Autodesk Inventor part; units mm, degrees
(part 2 of 4)
  spline S77 degree 3 poles (0.8273, -16.5454) (1.5125, -16.5454) (2.0682, -15.9899) (2.0682, -15.3045) knots 2 2 2 2 3 3 3 3
  line L679 (0.8273, -16.5454) -> (1.5125, -16.5454) construction
  line L680 (1.5125, -16.5454) -> (2.0682, -15.9899) construction
  line L681 (2.0682, -15.9899) -> (2.0682, -15.3045) construction
  line L682 (2.0682, -15.3045) -> (2.0682, -9.5136)
  spline S78 degree 3 poles (2.0682, -9.5136) (2.0682, -8.8282) (1.5125, -8.2727) (0.8273, -8.2727) knots 4 4 4 4 5 5 5 5
  line L683 (2.0682, -9.5136) -> (2.0682, -8.8282) construction
  line L684 (2.0682, -8.8282) -> (1.5125, -8.2727) construction
  line L685 (1.5125, -8.2727) -> (0.8273, -8.2727) construction
  line L686 (0.8273, -8.2727) -> (-0.8273, -8.2727)
  spline S79 degree 3 poles (-0.8273, -8.2727) (-1.5127, -8.2727) (-2.0682, -8.8282) (-2.0682, -9.5136) knots 6 6 6 6 7 7 7 7
  line L687 (-0.8273, -8.2727) -> (-1.5127, -8.2727) construction
  line L688 (-1.5127, -8.2727) -> (-2.0682, -8.8282) construction
  line L689 (-2.0682, -8.8282) -> (-2.0682, -9.5136) construction
  line L690 (-2.0682, -9.5136) -> (-2.0682, -15.3045)
  spline S80 degree 3 poles (-2.0682, -27.7134) (-2.0682, -28.399) (-1.5127, -28.9543) (-0.8273, -28.9543) knots 0 0 0 0 1 1 1 1
  line L691 (-2.0682, -27.7134) -> (-2.0682, -28.399) construction
  line L692 (-2.0682, -28.399) -> (-1.5127, -28.9543) construction
  line L693 (-1.5127, -28.9543) -> (-0.8273, -28.9543) construction
  line L694 (-0.8273, -28.9543) -> (0.8273, -28.9543)
  spline S81 degree 3 poles (0.8273, -28.9543) (1.5125, -28.9543) (2.0682, -28.399) (2.0682, -27.7134) knots 2 2 2 2 3 3 3 3
  line L695 (0.8273, -28.9543) -> (1.5125, -28.9543) construction
  line L696 (1.5125, -28.9543) -> (2.0682, -28.399) construction
  line L697 (2.0682, -28.399) -> (2.0682, -27.7134) construction
  line L698 (2.0682, -27.7134) -> (2.0682, -21.9225)
  spline S82 degree 3 poles (2.0682, -21.9225) (2.0682, -21.2373) (1.5125, -20.6816) (0.8273, -20.6816) knots 4 4 4 4 5 5 5 5
  line L699 (2.0682, -21.9225) -> (2.0682, -21.2373) construction
  line L700 (2.0682, -21.2373) -> (1.5125, -20.6816) construction
  line L701 (1.5125, -20.6816) -> (0.8273, -20.6816) construction
  line L702 (0.8273, -20.6816) -> (-0.8273, -20.6816)
  spline S83 degree 3 poles (-0.8273, -20.6816) (-1.5127, -20.6816) (-2.0682, -21.2373) (-2.0682, -21.9225) knots 6 6 6 6 7 7 7 7
  line L703 (-0.8273, -20.6816) -> (-1.5127, -20.6816) construction
  line L704 (-1.5127, -20.6816) -> (-2.0682, -21.2373) construction
  line L705 (-2.0682, -21.2373) -> (-2.0682, -21.9225) construction
  line L706 (-2.0682, -21.9225) -> (-2.0682, -27.7134)
  spline S84 degree 3 poles (-2.0682, -40.1226) (-2.0682, -40.8078) (-1.5127, -41.3635) (-0.8273, -41.3635) knots 0 0 0 0 1 1 1 1
  line L707 (-2.0682, -40.1226) -> (-2.0682, -40.8078) construction
  line L708 (-2.0682, -40.8078) -> (-1.5127, -41.3635) construction
  line L709 (-1.5127, -41.3635) -> (-0.8273, -41.3635) construction
  line L710 (-0.8273, -41.3635) -> (0.8273, -41.3635)
  spline S85 degree 3 poles (0.8273, -41.3635) (1.5125, -41.3635) (2.0682, -40.8078) (2.0682, -40.1226) knots 2 2 2 2 3 3 3 3
  line L711 (0.8273, -41.3635) -> (1.5125, -41.3635) construction
  line L712 (1.5125, -41.3635) -> (2.0682, -40.8078) construction
  line L713 (2.0682, -40.8078) -> (2.0682, -40.1226) construction
  line L714 (2.0682, -40.1226) -> (2.0682, -34.3318)
  spline S86 degree 3 poles (2.0682, -34.3318) (2.0682, -33.6462) (1.5125, -33.0908) (0.8273, -33.0908) knots 4 4 4 4 5 5 5 5
  line L715 (2.0682, -34.3318) -> (2.0682, -33.6462) construction
  line L716 (2.0682, -33.6462) -> (1.5125, -33.0908) construction
  line L717 (1.5125, -33.0908) -> (0.8273, -33.0908) construction
  line L718 (0.8273, -33.0908) -> (-0.8273, -33.0908)
  spline S87 degree 3 poles (-0.8273, -33.0908) (-1.5127, -33.0908) (-2.0682, -33.6462) (-2.0682, -34.3318) knots 6 6 6 6 7 7 7 7
  line L719 (-0.8273, -33.0908) -> (-1.5127, -33.0908) construction
  line L720 (-1.5127, -33.0908) -> (-2.0682, -33.6462) construction
  line L721 (-2.0682, -33.6462) -> (-2.0682, -34.3318) construction
  line L722 (-2.0682, -34.3318) -> (-2.0682, -40.1226)
  spline S88 degree 3 poles (-2.0682, -52.5315) (-2.0682, -53.2171) (-1.5127, -53.7724) (-0.8273, -53.7724) knots 0 0 0 0 1 1 1 1
  line L723 (-2.0682, -52.5315) -> (-2.0682, -53.2171) construction
  line L724 (-2.0682, -53.2171) -> (-1.5127, -53.7724) construction
  line L725 (-1.5127, -53.7724) -> (-0.8273, -53.7724) construction
  line L726 (-0.8273, -53.7724) -> (0.8273, -53.7724)
  spline S89 degree 3 poles (0.8273, -53.7724) (1.5125, -53.7724) (2.0682, -53.2171) (2.0682, -52.5315) knots 2 2 2 2 3 3 3 3
  line L727 (0.8273, -53.7724) -> (1.5125, -53.7724) construction
  line L728 (1.5125, -53.7724) -> (2.0682, -53.2171) construction
  line L729 (2.0682, -53.2171) -> (2.0682, -52.5315) construction
  line L730 (2.0682, -52.5315) -> (2.0682, -46.7406)
  spline S90 degree 3 poles (2.0682, -46.7406) (2.0682, -46.0554) (1.5125, -45.4997) (0.8273, -45.4997) knots 4 4 4 4 5 5 5 5
  line L731 (2.0682, -46.7406) -> (2.0682, -46.0554) construction
  line L732 (2.0682, -46.0554) -> (1.5125, -45.4997) construction
  line L733 (1.5125, -45.4997) -> (0.8273, -45.4997) construction
  line L734 (0.8273, -45.4997) -> (-0.8273, -45.4997)
  spline S91 degree 3 poles (-0.8273, -45.4997) (-1.5127, -45.4997) (-2.0682, -46.0554) (-2.0682, -46.7406) knots 6 6 6 6 7 7 7 7
  line L735 (-0.8273, -45.4997) -> (-1.5127, -45.4997) construction
  line L736 (-1.5127, -45.4997) -> (-2.0682, -46.0554) construction
  line L737 (-2.0682, -46.0554) -> (-2.0682, -46.7406) construction
  line L738 (-2.0682, -46.7406) -> (-2.0682, -52.5315)
  spline S92 degree 3 poles (-57.146, -14.6001) (-57.146, -13.3222) (-58.1819, -12.2864) (-59.4597, -12.2864) knots 0 0 0 0 1 1 1 1
  line L739 (-57.146, -14.6001) -> (-57.146, -13.3222) construction
  line L740 (-57.146, -13.3222) -> (-58.1819, -12.2864) construction
  line L741 (-58.1819, -12.2864) -> (-59.4597, -12.2864) construction
  line L742 (-59.4597, -12.2864) -> (-62.5446, -12.2864)
  spline S93 degree 3 poles (-62.5446, -12.2864) (-63.8225, -12.2864) (-64.8585, -13.3222) (-64.8585, -14.6001) knots 2 2 2 2 3 3 3 3
  line L743 (-62.5446, -12.2864) -> (-63.8225, -12.2864) construction
  line L744 (-63.8225, -12.2864) -> (-64.8585, -13.3222) construction
  line L745 (-64.8585, -13.3222) -> (-64.8585, -14.6001) construction
  line L746 (-64.8585, -14.6001) -> (-64.8585, -25.3976)
  spline S94 degree 3 poles (-64.8585, -25.3976) (-64.8585, -26.6754) (-63.8225, -27.7113) (-62.5446, -27.7113) knots 4 4 4 4 5 5 5 5
  line L747 (-64.8585, -25.3976) -> (-64.8585, -26.6754) construction
  line L748 (-64.8585, -26.6754) -> (-63.8225, -27.7113) construction
  line L749 (-63.8225, -27.7113) -> (-62.5446, -27.7113) construction
  line L750 (-62.5446, -27.7113) -> (-59.4597, -27.7113)
  spline S95 degree 3 poles (-59.4597, -27.7113) (-58.1819, -27.7113) (-57.146, -26.6754) (-57.146, -25.3976) knots 6 6 6 6 7 7 7 7
  line L751 (-59.4597, -27.7113) -> (-58.1819, -27.7113) construction
  line L752 (-58.1819, -27.7113) -> (-57.146, -26.6754) construction
  line L753 (-57.146, -26.6754) -> (-57.146, -25.3976) construction
  line L754 (-57.146, -25.3976) -> (-57.146, -14.6001)
  spline S96 degree 3 poles (-57.146, 5.3998) (-57.146, 6.6778) (-58.1819, 7.7136) (-59.4597, 7.7136) knots 0 0 0 0 1 1 1 1
  line L755 (-57.146, 5.3998) -> (-57.146, 6.6778) construction
  line L756 (-57.146, 6.6778) -> (-58.1819, 7.7136) construction
  line L757 (-58.1819, 7.7136) -> (-59.4597, 7.7136) construction
  line L758 (-59.4597, 7.7136) -> (-62.5446, 7.7136)
  spline S97 degree 3 poles (-62.5446, 7.7136) (-63.8225, 7.7136) (-64.8585, 6.6778) (-64.8585, 5.3998) knots 2 2 2 2 3 3 3 3
  line L759 (-62.5446, 7.7136) -> (-63.8225, 7.7136) construction
  line L760 (-63.8225, 7.7136) -> (-64.8585, 6.6778) construction
  line L761 (-64.8585, 6.6778) -> (-64.8585, 5.3998) construction
  line L762 (-64.8585, 5.3998) -> (-64.8585, -5.3976)
  spline S98 degree 3 poles (-64.8585, -5.3976) (-64.8585, -6.6756) (-63.8225, -7.7113) (-62.5446, -7.7113) knots 4 4 4 4 5 5 5 5
  line L763 (-64.8585, -5.3976) -> (-64.8585, -6.6756) construction
  line L764 (-64.8585, -6.6756) -> (-63.8225, -7.7113) construction
  line L765 (-63.8225, -7.7113) -> (-62.5446, -7.7113) construction
  line L766 (-62.5446, -7.7113) -> (-59.4597, -7.7113)
  spline S99 degree 3 poles (-59.4597, -7.7113) (-58.1819, -7.7113) (-57.146, -6.6756) (-57.146, -5.3976) knots 6 6 6 6 7 7 7 7
  line L767 (-59.4597, -7.7113) -> (-58.1819, -7.7113) construction
  line L768 (-58.1819, -7.7113) -> (-57.146, -6.6756) construction
  line L769 (-57.146, -6.6756) -> (-57.146, -5.3976) construction
  line L770 (-57.146, -5.3976) -> (-57.146, 5.3998)
  spline S100 degree 3 poles (-57.146, 25.3998) (-57.146, 26.6778) (-58.1819, 27.7137) (-59.4597, 27.7137) knots 0 0 0 0 1 1 1 1
  line L771 (-57.146, 25.3998) -> (-57.146, 26.6778) construction
  line L772 (-57.146, 26.6778) -> (-58.1819, 27.7137) construction
  line L773 (-58.1819, 27.7137) -> (-59.4597, 27.7137) construction
  line L774 (-59.4597, 27.7137) -> (-62.5446, 27.7137)
  spline S101 degree 3 poles (-62.5446, 27.7137) (-63.8225, 27.7137) (-64.8585, 26.6778) (-64.8585, 25.3998) knots 2 2 2 2 3 3 3 3
  line L775 (-62.5446, 27.7137) -> (-63.8225, 27.7137) construction
  line L776 (-63.8225, 27.7137) -> (-64.8585, 26.6778) construction
  line L777 (-64.8585, 26.6778) -> (-64.8585, 25.3998) construction
  line L778 (-64.8585, 25.3998) -> (-64.8585, 14.6024)
  spline S102 degree 3 poles (-64.8585, 14.6024) (-64.8585, 13.3246) (-63.8225, 12.2887) (-62.5446, 12.2887) knots 4 4 4 4 5 5 5 5
  line L779 (-64.8585, 14.6024) -> (-64.8585, 13.3246) construction
  line L780 (-64.8585, 13.3246) -> (-63.8225, 12.2887) construction
  line L781 (-63.8225, 12.2887) -> (-62.5446, 12.2887) construction
  line L782 (-62.5446, 12.2887) -> (-59.4597, 12.2887)
  spline S103 degree 3 poles (-59.4597, 12.2887) (-58.1819, 12.2887) (-57.146, 13.3246) (-57.146, 14.6024) knots 6 6 6 6 7 7 7 7
  line L783 (-59.4597, 12.2887) -> (-58.1819, 12.2887) construction
  line L784 (-58.1819, 12.2887) -> (-57.146, 13.3246) construction
  line L785 (-57.146, 13.3246) -> (-57.146, 14.6024) construction
  line L786 (-57.146, 14.6024) -> (-57.146, 25.3998)
  spline S104 degree 3 poles (64.8562, -14.6001) (64.8562, -13.3222) (63.8203, -12.2864) (62.5422, -12.2864) knots 0 0 0 0 1 1 1 1
  line L787 (64.8562, -14.6001) -> (64.8562, -13.3222) construction
  line L788 (64.8562, -13.3222) -> (63.8203, -12.2864) construction
  line L789 (63.8203, -12.2864) -> (62.5422, -12.2864) construction
  line L790 (62.5422, -12.2864) -> (59.4574, -12.2864)
  spline S105 degree 3 poles (59.4574, -12.2864) (58.1797, -12.2864) (57.1437, -13.3222) (57.1437, -14.6001) knots 2 2 2 2 3 3 3 3
  line L791 (59.4574, -12.2864) -> (58.1797, -12.2864) construction
  line L792 (58.1797, -12.2864) -> (57.1437, -13.3222) construction
  line L793 (57.1437, -13.3222) -> (57.1437, -14.6001) construction
  line L794 (57.1437, -14.6001) -> (57.1437, -25.3976)
  spline S106 degree 3 poles (57.1437, -25.3976) (57.1437, -26.6754) (58.1797, -27.7113) (59.4574, -27.7113) knots 4 4 4 4 5 5 5 5
  line L795 (57.1437, -25.3976) -> (57.1437, -26.6754) construction
  line L796 (57.1437, -26.6754) -> (58.1797, -27.7113) construction
  line L797 (58.1797, -27.7113) -> (59.4574, -27.7113) construction
  line L798 (59.4574, -27.7113) -> (62.5422, -27.7113)
  spline S107 degree 3 poles (62.5422, -27.7113) (63.8203, -27.7113) (64.8562, -26.6754) (64.8562, -25.3976) knots 6 6 6 6 7 7 7 7
  line L799 (62.5422, -27.7113) -> (63.8203, -27.7113) construction
  line L800 (63.8203, -27.7113) -> (64.8562, -26.6754) construction
  line L801 (64.8562, -26.6754) -> (64.8562, -25.3976) construction
  line L802 (64.8562, -25.3976) -> (64.8562, -14.6001)
  spline S108 degree 3 poles (64.8562, 5.3998) (64.8562, 6.6778) (63.8203, 7.7136) (62.5422, 7.7136) knots 0 0 0 0 1 1 1 1
  line L803 (64.8562, 5.3998) -> (64.8562, 6.6778) construction
  line L804 (64.8562, 6.6778) -> (63.8203, 7.7136) construction
  line L805 (63.8203, 7.7136) -> (62.5422, 7.7136) construction
  line L806 (62.5422, 7.7136) -> (59.4574, 7.7136)
  spline S109 degree 3 poles (59.4574, 7.7136) (58.1797, 7.7136) (57.1437, 6.6778) (57.1437, 5.3998) knots 2 2 2 2 3 3 3 3
  line L807 (59.4574, 7.7136) -> (58.1797, 7.7136) construction
  line L808 (58.1797, 7.7136) -> (57.1437, 6.6778) construction
  line L809 (57.1437, 6.6778) -> (57.1437, 5.3998) construction
  line L810 (57.1437, 5.3998) -> (57.1437, -5.3976)
  spline S110 degree 3 poles (57.1437, -5.3976) (57.1437, -6.6756) (58.1797, -7.7113) (59.4574, -7.7113) knots 4 4 4 4 5 5 5 5
  line L811 (57.1437, -5.3976) -> (57.1437, -6.6756) construction
  line L812 (57.1437, -6.6756) -> (58.1797, -7.7113) construction
  line L813 (58.1797, -7.7113) -> (59.4574, -7.7113) construction
  line L814 (59.4574, -7.7113) -> (62.5422, -7.7113)
  spline S111 degree 3 poles (62.5422, -7.7113) (63.8203, -7.7113) (64.8562, -6.6756) (64.8562, -5.3976) knots 6 6 6 6 7 7 7 7
  line L815 (62.5422, -7.7113) -> (63.8203, -7.7113) construction
  line L816 (63.8203, -7.7113) -> (64.8562, -6.6756) construction
  line L817 (64.8562, -6.6756) -> (64.8562, -5.3976) construction
  line L818 (64.8562, -5.3976) -> (64.8562, 5.3998)
  spline S112 degree 3 poles (64.8562, 25.3998) (64.8562, 26.6778) (63.8203, 27.7137) (62.5422, 27.7137) knots 0 0 0 0 1 1 1 1
  line L819 (64.8562, 25.3998) -> (64.8562, 26.6778) construction
  line L820 (64.8562, 26.6778) -> (63.8203, 27.7137) construction
  line L821 (63.8203, 27.7137) -> (62.5422, 27.7137) construction
  line L822 (62.5422, 27.7137) -> (59.4574, 27.7137)
  spline S113 degree 3 poles (59.4574, 27.7137) (58.1797, 27.7137) (57.1437, 26.6778) (57.1437, 25.3998) knots 2 2 2 2 3 3 3 3
  line L823 (59.4574, 27.7137) -> (58.1797, 27.7137) construction
  line L824 (58.1797, 27.7137) -> (57.1437, 26.6778) construction
  line L825 (57.1437, 26.6778) -> (57.1437, 25.3998) construction
  line L826 (57.1437, 25.3998) -> (57.1437, 14.6024)
  spline S114 degree 3 poles (57.1437, 14.6024) (57.1437, 13.3246) (58.1797, 12.2887) (59.4574, 12.2887) knots 4 4 4 4 5 5 5 5
  line L827 (57.1437, 14.6024) -> (57.1437, 13.3246) construction
  line L828 (57.1437, 13.3246) -> (58.1797, 12.2887) construction
  line L829 (58.1797, 12.2887) -> (59.4574, 12.2887) construction
  line L830 (59.4574, 12.2887) -> (62.5422, 12.2887)
  spline S115 degree 3 poles (62.5422, 12.2887) (63.8203, 12.2887) (64.8562, 13.3246) (64.8562, 14.6024) knots 6 6 6 6 7 7 7 7
  line L831 (62.5422, 12.2887) -> (63.8203, 12.2887) construction
  line L832 (63.8203, 12.2887) -> (64.8562, 13.3246) construction
  line L833 (64.8562, 13.3246) -> (64.8562, 14.6024) construction
  line L834 (64.8562, 14.6024) -> (64.8562, 25.3998)
  spline S116 degree 3 poles (-48.9787, 43.5169) (-49.8823, 44.4205) (-49.8823, 45.8856) (-48.9787, 46.789) knots 0 0 0 0 1 1 1 1
  line L835 (-48.9787, 43.5169) -> (-49.8823, 44.4205) construction
  line L836 (-49.8823, 44.4205) -> (-49.8823, 45.8856) construction
  line L837 (-49.8823, 45.8856) -> (-48.9787, 46.789) construction
  line L838 (-48.9787, 46.789) -> (-46.7972, 48.9705)
  spline S117 degree 3 poles (-46.7972, 48.9705) (-45.8938, 49.8741) (-44.4287, 49.8741) (-43.5253, 48.9705) knots 2 2 2 2 3 3 3 3
  line L839 (-46.7972, 48.9705) -> (-45.8938, 49.8741) construction
  line L840 (-45.8938, 49.8741) -> (-44.4287, 49.8741) construction
  line L841 (-44.4287, 49.8741) -> (-43.5253, 48.9705) construction
  line L842 (-43.5253, 48.9705) -> (-35.8902, 41.3355)
  spline S118 degree 3 poles (-35.8902, 41.3355) (-34.9866, 40.432) (-34.9866, 38.967) (-35.8902, 38.0633) knots 4 4 4 4 5 5 5 5
  line L843 (-35.8902, 41.3355) -> (-34.9866, 40.432) construction
  line L844 (-34.9866, 40.432) -> (-34.9866, 38.967) construction
  line L845 (-34.9866, 38.967) -> (-35.8902, 38.0633) construction
  line L846 (-35.8902, 38.0633) -> (-38.0717, 35.882)
  spline S119 degree 3 poles (-38.0717, 35.882) (-38.9751, 34.9784) (-40.4402, 34.9784) (-41.3438, 35.882) knots 6 6 6 6 7 7 7 7
  line L847 (-38.0717, 35.882) -> (-38.9751, 34.9784) construction
  line L848 (-38.9751, 34.9784) -> (-40.4402, 34.9784) construction
  line L849 (-40.4402, 34.9784) -> (-41.3438, 35.882) construction
  line L850 (-41.3438, 35.882) -> (-48.9787, 43.5169)
  spline S120 degree 3 poles (-34.8365, 29.3748) (-35.7402, 30.2784) (-35.7402, 31.7435) (-34.8365, 32.6469) knots 0 0 0 0 1 1 1 1
  line L851 (-34.8365, 29.3748) -> (-35.7402, 30.2784) construction
  line L852 (-35.7402, 30.2784) -> (-35.7402, 31.7435) construction
  line L853 (-35.7402, 31.7435) -> (-34.8365, 32.6469) construction
  line L854 (-34.8365, 32.6469) -> (-32.6551, 34.8284)
  spline S121 degree 3 poles (-32.6551, 34.8284) (-31.7516, 35.732) (-30.2866, 35.732) (-29.383, 34.8284) knots 2 2 2 2 3 3 3 3
  line L855 (-32.6551, 34.8284) -> (-31.7516, 35.732) construction
  line L856 (-31.7516, 35.732) -> (-30.2866, 35.732) construction
  line L857 (-30.2866, 35.732) -> (-29.383, 34.8284) construction
  line L858 (-29.383, 34.8284) -> (-21.7481, 27.1933)
  spline S122 degree 3 poles (-21.7481, 27.1933) (-20.8445, 26.2899) (-20.8445, 24.8248) (-21.7481, 23.9212) knots 4 4 4 4 5 5 5 5
  line L859 (-21.7481, 27.1933) -> (-20.8445, 26.2899) construction
  line L860 (-20.8445, 26.2899) -> (-20.8445, 24.8248) construction
  line L861 (-20.8445, 24.8248) -> (-21.7481, 23.9212) construction
  line L862 (-21.7481, 23.9212) -> (-23.9295, 21.7398)
  spline S123 degree 3 poles (-23.9295, 21.7398) (-24.833, 20.8363) (-26.2981, 20.8363) (-27.2015, 21.7398) knots 6 6 6 6 7 7 7 7
  line L863 (-23.9295, 21.7398) -> (-24.833, 20.8363) construction
  line L864 (-24.833, 20.8363) -> (-26.2981, 20.8363) construction
  line L865 (-26.2981, 20.8363) -> (-27.2015, 21.7398) construction
  line L866 (-27.2015, 21.7398) -> (-34.8365, 29.3748)
  spline S124 degree 3 poles (-20.6944, 15.2327) (-21.5981, 16.1363) (-21.5981, 17.6013) (-20.6944, 18.5048) knots 0 0 0 0 1 1 1 1
  line L867 (-20.6944, 15.2327) -> (-21.5981, 16.1363) construction
  line L868 (-21.5981, 16.1363) -> (-21.5981, 17.6013) construction
  line L869 (-21.5981, 17.6013) -> (-20.6944, 18.5048) construction
  line L870 (-20.6944, 18.5048) -> (-18.513, 20.6862)
  spline S125 degree 3 poles (-18.513, 20.6862) (-17.6095, 21.5899) (-16.1445, 21.5899) (-15.2408, 20.6862) knots 2 2 2 2 3 3 3 3
  line L871 (-18.513, 20.6862) -> (-17.6095, 21.5899) construction
  line L872 (-17.6095, 21.5899) -> (-16.1445, 21.5899) construction
  line L873 (-16.1445, 21.5899) -> (-15.2408, 20.6862) construction
  line L874 (-15.2408, 20.6862) -> (-7.6058, 13.0512)
  spline S126 degree 3 poles (-7.6058, 13.0512) (-6.7023, 12.1478) (-6.7023, 10.6827) (-7.6058, 9.7791) knots 4 4 4 4 5 5 5 5
  line L875 (-7.6058, 13.0512) -> (-6.7023, 12.1478) construction
  line L876 (-6.7023, 12.1478) -> (-6.7023, 10.6827) construction
  line L877 (-6.7023, 10.6827) -> (-7.6058, 9.7791) construction
  line L878 (-7.6058, 9.7791) -> (-9.7873, 7.5976)
  spline S127 degree 3 poles (-9.7873, 7.5976) (-10.6909, 6.6942) (-12.1559, 6.6942) (-13.0594, 7.5976) knots 6 6 6 6 7 7 7 7
  line L879 (-9.7873, 7.5976) -> (-10.6909, 6.6942) construction
  line L880 (-10.6909, 6.6942) -> (-12.1559, 6.6942) construction
  line L881 (-12.1559, 6.6942) -> (-13.0594, 7.5976) construction
  line L882 (-13.0594, 7.5976) -> (-20.6944, 15.2327)
  spline S128 degree 3 poles (7.5898, -13.0516) (6.6862, -12.1481) (6.6862, -10.6831) (7.5898, -9.7794) knots 0 0 0 0 1 1 1 1
  line L883 (7.5898, -13.0516) -> (6.6862, -12.1481) construction
  line L884 (6.6862, -12.1481) -> (6.6862, -10.6831) construction
  line L885 (6.6862, -10.6831) -> (7.5898, -9.7794) construction
  line L886 (7.5898, -9.7794) -> (9.7712, -7.598)
  spline S129 degree 3 poles (9.7712, -7.598) (10.6749, -6.6945) (12.1397, -6.6945) (13.0434, -7.598) knots 2 2 2 2 3 3 3 3
  line L887 (9.7712, -7.598) -> (10.6749, -6.6945) construction
  line L888 (10.6749, -6.6945) -> (12.1397, -6.6945) construction
  line L889 (12.1397, -6.6945) -> (13.0434, -7.598) construction
  line L890 (13.0434, -7.598) -> (20.6784, -15.233)
  spline S130 degree 3 poles (20.6784, -15.233) (21.5821, -16.1367) (21.5821, -17.6015) (20.6784, -18.505) knots 4 4 4 4 5 5 5 5
  line L891 (20.6784, -15.233) -> (21.5821, -16.1367) construction
  line L892 (21.5821, -16.1367) -> (21.5821, -17.6015) construction
  line L893 (21.5821, -17.6015) -> (20.6784, -18.505) construction
  line L894 (20.6784, -18.505) -> (18.497, -20.6864)
  spline S131 degree 3 poles (18.497, -20.6864) (17.5933, -21.5901) (16.1285, -21.5901) (15.2248, -20.6864) knots 6 6 6 6 7 7 7 7
  line L895 (18.497, -20.6864) -> (17.5933, -21.5901) construction
  line L896 (17.5933, -21.5901) -> (16.1285, -21.5901) construction
  line L897 (16.1285, -21.5901) -> (15.2248, -20.6864) construction
  line L898 (15.2248, -20.6864) -> (7.5898, -13.0516)
  line L899 (27.6826, -22.255) -> (26.9926, -21.5649)
  spline S132 degree 3 poles (26.9926, -21.5649) (26.0958, -20.6682) (24.642, -20.6682) (23.7452, -21.5649) knots 1 1 1 1 2 2 2 2
  line L900 (26.9926, -21.5649) -> (26.0958, -20.6682) construction
  line L901 (26.0958, -20.6682) -> (24.642, -20.6682) construction
  line L902 (24.642, -20.6682) -> (23.7452, -21.5649) construction
  line L903 (23.7452, -21.5649) -> (21.58, -23.7298)
  spline S133 degree 3 poles (21.58, -23.7298) (20.6832, -24.6269) (20.6832, -26.0808) (21.58, -26.9775) knots 3 3 3 3 4 4 4 4
  line L904 (21.58, -23.7298) -> (20.6832, -24.6269) construction
  line L905 (20.6832, -24.6269) -> (20.6832, -26.0808) construction
  line L906 (20.6832, -26.0808) -> (21.58, -26.9775) construction
  line L907 (21.58, -26.9775) -> (22.27, -27.6676)
  line L908 (22.27, -27.6676) -> (24.2024, -29.5999)
  spline S134 degree 3 poles (24.2024, -29.5999) (25.0992, -30.4967) (26.553, -30.4967) (27.4497, -29.5999) knots 6 6 6 6 7 7 7 7
  line L909 (24.2024, -29.5999) -> (25.0992, -30.4967) construction
  line L910 (25.0992, -30.4967) -> (26.553, -30.4967) construction
  line L911 (26.553, -30.4967) -> (27.4497, -29.5999) construction
  line L912 (27.4497, -29.5999) -> (29.615, -27.4347)
  spline S135 degree 3 poles (29.615, -27.4347) (30.5117, -26.5379) (30.5117, -25.0841) (29.615, -24.1873) knots 8 8 8 8 9 9 9 9
  line L913 (29.615, -27.4347) -> (30.5117, -26.5379) construction
  line L914 (30.5117, -26.5379) -> (30.5117, -25.0841) construction
  line L915 (30.5117, -25.0841) -> (29.615, -24.1873) construction
  line L916 (29.615, -24.1873) -> (27.6826, -22.255)
  line L917 (32.9616, -34.5977) -> (32.7521, -34.5874)
  line L918 (32.7521, -34.5874) -> (32.5485, -34.5564)
  line L919 (32.5485, -34.5564) -> (32.3521, -34.5057)
  line L920 (32.3521, -34.5057) -> (32.1637, -34.4368)
  line L921 (32.1637, -34.4368) -> (31.9845, -34.3504)
  line L922 (31.9845, -34.3504) -> (31.8154, -34.2477)
  line L923 (31.8154, -34.2477) -> (31.6576, -34.1299)
  line L924 (31.6576, -34.1299) -> (31.5122, -33.9976)
  line L925 (31.5122, -33.9976) -> (31.3796, -33.8519)
  line L926 (31.3796, -33.8519) -> (31.2617, -33.6941)
  line L927 (31.2617, -33.6941) -> (31.1591, -33.5249)
  line L928 (31.1591, -33.5249) -> (31.0726, -33.3458)
  line L929 (31.0726, -33.3458) -> (31.0037, -33.1573)
  line L930 (31.0037, -33.1573) -> (30.9534, -32.961)
  line L931 (30.9534, -32.961) -> (30.9221, -32.7573)
  line L932 (30.9221, -32.7573) -> (30.9117, -32.5479)
  line L933 (30.9117, -32.5479) -> (30.9221, -32.3384)
  line L934 (30.9221, -32.3384) -> (30.9534, -32.1348)
  line L935 (30.9534, -32.1348) -> (31.0037, -31.9381)
  line L936 (31.0037, -31.9381) -> (31.0726, -31.75)
  line L937 (31.0726, -31.75) -> (31.1591, -31.5709)
  line L938 (31.1591, -31.5709) -> (31.2617, -31.4017)
  line L939 (31.2617, -31.4017) -> (31.3796, -31.2439)
  line L940 (31.3796, -31.2439) -> (31.5122, -31.0982)
  line L941 (31.5122, -31.0982) -> (31.6576, -30.9659)
  line L942 (31.6576, -30.9659) -> (31.8154, -30.8481)
  line L943 (31.8154, -30.8481) -> (31.9845, -30.7454)
  line L944 (31.9845, -30.7454) -> (32.1637, -30.6589)
  line L945 (32.1637, -30.6589) -> (32.3521, -30.59)
  line L946 (32.3521, -30.59) -> (32.5485, -30.5394)
  line L947 (32.5485, -30.5394) -> (32.7521, -30.5084)
  line L948 (32.7521, -30.5084) -> (32.9616, -30.4977)
  line L949 (32.9616, -30.4977) -> (33.1714, -30.5084)
  line L950 (33.1714, -30.5084) -> (33.3746, -30.5394)
  line L951 (33.3746, -30.5394) -> (33.5713, -30.59)
  line L952 (33.5713, -30.59) -> (33.7594, -30.6589)
  line L953 (33.7594, -30.6589) -> (33.9389, -30.7454)
  line L954 (33.9389, -30.7454) -> (34.1077, -30.8481)
  line L955 (34.1077, -30.8481) -> (34.2655, -30.9659)
  line L956 (34.2655, -30.9659) -> (34.4113, -31.0982)
  line L957 (34.4113, -31.0982) -> (34.5435, -31.2439)
  line L958 (34.5435, -31.2439) -> (34.6614, -31.4017)
  line L959 (34.6614, -31.4017) -> (34.764, -31.5709)
  line L960 (34.764, -31.5709) -> (34.8505, -31.75)
  line L961 (34.8505, -31.75) -> (34.9194, -31.9381)
  line L962 (34.9194, -31.9381) -> (34.97, -32.1348)
  line L963 (34.97, -32.1348) -> (35.0011, -32.3384)
  line L964 (35.0011, -32.3384) -> (35.0117, -32.5479)
  line L965 (35.0117, -32.5479) -> (35.0011, -32.7573)
  line L966 (35.0011, -32.7573) -> (34.97, -32.961)
  line L967 (34.97, -32.961) -> (34.9194, -33.1573)
  line L968 (34.9194, -33.1573) -> (34.8505, -33.3458)
  line L969 (34.8505, -33.3458) -> (34.764, -33.5249)
  line L970 (34.764, -33.5249) -> (34.6614, -33.6941)
  line L971 (34.6614, -33.6941) -> (34.5435, -33.8519)
  line L972 (34.5435, -33.8519) -> (34.4113, -33.9976)
  line L973 (34.4113, -33.9976) -> (34.2655, -34.1299)
  line L974 (34.2655, -34.1299) -> (34.1077, -34.2477)
  line L975 (34.1077, -34.2477) -> (33.9389, -34.3504)
  line L976 (33.9389, -34.3504) -> (33.7594, -34.4368)
  line L977 (33.7594, -34.4368) -> (33.5713, -34.5057)
  line L978 (33.5713, -34.5057) -> (33.3746, -34.5564)
  line L979 (33.3746, -34.5564) -> (33.1714, -34.5874)
  line L980 (33.1714, -34.5874) -> (32.9616, -34.5977)
  spline S136 degree 3 poles (35.874, -41.336) (34.9704, -40.4323) (34.9704, -38.9671) (35.874, -38.0638) knots 0 0 0 0 1 1 1 1
  line L981 (35.874, -41.336) -> (34.9704, -40.4323) construction
  line L982 (34.9704, -40.4323) -> (34.9704, -38.9671) construction
  line L983 (34.9704, -38.9671) -> (35.874, -38.0638) construction
  line L984 (35.874, -38.0638) -> (38.0555, -35.8824)
  spline S137 degree 3 poles (38.0555, -35.8824) (38.9591, -34.9787) (40.424, -34.9787) (41.3276, -35.8824) knots 2 2 2 2 3 3 3 3
  line L985 (38.0555, -35.8824) -> (38.9591, -34.9787) construction
  line L986 (38.9591, -34.9787) -> (40.424, -34.9787) construction
  line L987 (40.424, -34.9787) -> (41.3276, -35.8824) construction
  line L988 (41.3276, -35.8824) -> (48.9626, -43.5174)
  spline S138 degree 3 poles (48.9626, -43.5174) (49.8663, -44.4207) (49.8663, -45.8859) (48.9626, -46.7896) knots 4 4 4 4 5 5 5 5
  line L989 (48.9626, -43.5174) -> (49.8663, -44.4207) construction
  line L990 (49.8663, -44.4207) -> (49.8663, -45.8859) construction
  line L991 (49.8663, -45.8859) -> (48.9626, -46.7896) construction
  line L992 (48.9626, -46.7896) -> (46.7812, -48.971)
  spline S139 degree 3 poles (46.7812, -48.971) (45.8776, -49.8743) (44.4127, -49.8743) (43.5091, -48.971) knots 6 6 6 6 7 7 7 7
  line L993 (46.7812, -48.971) -> (45.8776, -49.8743) construction
  line L994 (45.8776, -49.8743) -> (44.4127, -49.8743) construction
  line L995 (44.4127, -49.8743) -> (43.5091, -48.971) construction
  line L996 (43.5091, -48.971) -> (35.874, -41.336)
  spline S140 degree 3 poles (-35.8902, -41.336) (-34.9866, -40.4323) (-34.9866, -38.9671) (-35.8902, -38.0638) knots 0 0 0 0 1 1 1 1
  line L997 (-35.8902, -41.336) -> (-34.9866, -40.4323) construction
  line L998 (-34.9866, -40.4323) -> (-34.9866, -38.9671) construction
  line L999 (-34.9866, -38.9671) -> (-35.8902, -38.0638) construction
  line L1000 (-35.8902, -38.0638) -> (-38.0717, -35.8824)
  spline S141 degree 3 poles (-38.0717, -35.8824) (-38.9751, -34.9787) (-40.4402, -34.9787) (-41.3438, -35.8824) knots 2 2 2 2 3 3 3 3
  line L1001 (-38.0717, -35.8824) -> (-38.9751, -34.9787) construction
  line L1002 (-38.9751, -34.9787) -> (-40.4402, -34.9787) construction
  line L1003 (-40.4402, -34.9787) -> (-41.3438, -35.8824) construction
  line L1004 (-41.3438, -35.8824) -> (-48.9787, -43.5174)
  spline S142 degree 3 poles (-48.9787, -43.5174) (-49.8823, -44.4207) (-49.8823, -45.8859) (-48.9787, -46.7896) knots 4 4 4 4 5 5 5 5
  line L1005 (-48.9787, -43.5174) -> (-49.8823, -44.4207) construction
  line L1006 (-49.8823, -44.4207) -> (-49.8823, -45.8859) construction
  line L1007 (-49.8823, -45.8859) -> (-48.9787, -46.7896) construction
  line L1008 (-48.9787, -46.7896) -> (-46.7972, -48.971)
  spline S143 degree 3 poles (-46.7972, -48.971) (-45.8938, -49.8743) (-44.4287, -49.8743) (-43.5253, -48.971) knots 6 6 6 6 7 7 7 7
  line L1009 (-46.7972, -48.971) -> (-45.8938, -49.8743) construction
  line L1010 (-45.8938, -49.8743) -> (-44.4287, -49.8743) construction
  line L1011 (-44.4287, -49.8743) -> (-43.5253, -48.971) construction
  line L1012 (-43.5253, -48.971) -> (-35.8902, -41.336)
  spline S144 degree 3 poles (-21.7481, -27.1939) (-20.8445, -26.2902) (-20.8445, -24.825) (-21.7481, -23.9217) knots 0 0 0 0 1 1 1 1
  line L1013 (-21.7481, -27.1939) -> (-20.8445, -26.2902) construction
  line L1014 (-20.8445, -26.2902) -> (-20.8445, -24.825) construction
  line L1015 (-20.8445, -24.825) -> (-21.7481, -23.9217) construction
  line L1016 (-21.7481, -23.9217) -> (-23.9295, -21.7403)
  spline S145 degree 3 poles (-23.9295, -21.7403) (-24.833, -20.8366) (-26.2981, -20.8366) (-27.2015, -21.7403) knots 2 2 2 2 3 3 3 3
  line L1017 (-23.9295, -21.7403) -> (-24.833, -20.8366) construction
  line L1018 (-24.833, -20.8366) -> (-26.2981, -20.8366) construction
  line L1019 (-26.2981, -20.8366) -> (-27.2015, -21.7403) construction
  line L1020 (-27.2015, -21.7403) -> (-34.8365, -29.3753)
  spline S146 degree 3 poles (-34.8365, -29.3753) (-35.7402, -30.2786) (-35.7402, -31.7438) (-34.8365, -32.6474) knots 4 4 4 4 5 5 5 5
  line L1021 (-34.8365, -29.3753) -> (-35.7402, -30.2786) construction
  line L1022 (-35.7402, -30.2786) -> (-35.7402, -31.7438) construction
  line L1023 (-35.7402, -31.7438) -> (-34.8365, -32.6474) construction
  line L1024 (-34.8365, -32.6474) -> (-32.6551, -34.8289)
  spline S147 degree 3 poles (-32.6551, -34.8289) (-31.7516, -35.7322) (-30.2866, -35.7322) (-29.383, -34.8289) knots 6 6 6 6 7 7 7 7
  line L1025 (-32.6551, -34.8289) -> (-31.7516, -35.7322) construction
  line L1026 (-31.7516, -35.7322) -> (-30.2866, -35.7322) construction
  line L1027 (-30.2866, -35.7322) -> (-29.383, -34.8289) construction
  line L1028 (-29.383, -34.8289) -> (-21.7481, -27.1939)
  spline S148 degree 3 poles (-7.6058, -13.0516) (-6.7023, -12.1481) (-6.7023, -10.6831) (-7.6058, -9.7794) knots 0 0 0 0 1 1 1 1
  line L1029 (-7.6058, -13.0516) -> (-6.7023, -12.1481) construction
  line L1030 (-6.7023, -12.1481) -> (-6.7023, -10.6831) construction
  line L1031 (-6.7023, -10.6831) -> (-7.6058, -9.7794) construction
  line L1032 (-7.6058, -9.7794) -> (-9.7873, -7.598)
  spline S149 degree 3 poles (-9.7873, -7.598) (-10.6909, -6.6945) (-12.1559, -6.6945) (-13.0594, -7.598) knots 2 2 2 2 3 3 3 3
  line L1033 (-9.7873, -7.598) -> (-10.6909, -6.6945) construction
  line L1034 (-10.6909, -6.6945) -> (-12.1559, -6.6945) construction
  line L1035 (-12.1559, -6.6945) -> (-13.0594, -7.598) construction
  line L1036 (-13.0594, -7.598) -> (-20.6944, -15.233)
  spline S150 degree 3 poles (-20.6944, -15.233) (-21.5981, -16.1367) (-21.5981, -17.6015) (-20.6944, -18.505) knots 4 4 4 4 5 5 5 5
  line L1037 (-20.6944, -15.233) -> (-21.5981, -16.1367) construction
  line L1038 (-21.5981, -16.1367) -> (-21.5981, -17.6015) construction
  line L1039 (-21.5981, -17.6015) -> (-20.6944, -18.505) construction
  line L1040 (-20.6944, -18.505) -> (-18.513, -20.6864)
  spline S151 degree 3 poles (-18.513, -20.6864) (-17.6095, -21.5901) (-16.1445, -21.5901) (-15.2408, -20.6864) knots 6 6 6 6 7 7 7 7
  line L1041 (-18.513, -20.6864) -> (-17.6095, -21.5901) construction
  line L1042 (-17.6095, -21.5901) -> (-16.1445, -21.5901) construction
  line L1043 (-16.1445, -21.5901) -> (-15.2408, -20.6864) construction
  line L1044 (-15.2408, -20.6864) -> (-7.6058, -13.0516)
  spline S152 degree 3 poles (20.6784, 15.2327) (21.5821, 16.1363) (21.5821, 17.6013) (20.6784, 18.5048) knots 0 0 0 0 1 1 1 1
  line L1045 (20.6784, 15.2327) -> (21.5821, 16.1363) construction
  line L1046 (21.5821, 16.1363) -> (21.5821, 17.6013) construction
  line L1047 (21.5821, 17.6013) -> (20.6784, 18.5048) construction
  line L1048 (20.6784, 18.5048) -> (18.497, 20.6862)
  spline S153 degree 3 poles (18.497, 20.6862) (17.5933, 21.5899) (16.1285, 21.5899) (15.2248, 20.6862) knots 2 2 2 2 3 3 3 3
  line L1049 (18.497, 20.6862) -> (17.5933, 21.5899) construction
  line L1050 (17.5933, 21.5899) -> (16.1285, 21.5899) construction
  line L1051 (16.1285, 21.5899) -> (15.2248, 20.6862) construction
  line L1052 (15.2248, 20.6862) -> (7.5898, 13.0512)
  spline S154 degree 3 poles (7.5898, 13.0512) (6.6862, 12.1478) (6.6862, 10.6827) (7.5898, 9.7791) knots 4 4 4 4 5 5 5 5
  line L1053 (7.5898, 13.0512) -> (6.6862, 12.1478) construction
  line L1054 (6.6862, 12.1478) -> (6.6862, 10.6827) construction
  line L1055 (6.6862, 10.6827) -> (7.5898, 9.7791) construction
  line L1056 (7.5898, 9.7791) -> (9.7712, 7.5976)
  spline S155 degree 3 poles (9.7712, 7.5976) (10.6749, 6.6942) (12.1397, 6.6942) (13.0434, 7.5976) knots 6 6 6 6 7 7 7 7
  line L1057 (9.7712, 7.5976) -> (10.6749, 6.6942) construction
  line L1058 (10.6749, 6.6942) -> (12.1397, 6.6942) construction
  line L1059 (12.1397, 6.6942) -> (13.0434, 7.5976) construction
  line L1060 (13.0434, 7.5976) -> (20.6784, 15.2327)
  spline S156 degree 3 poles (34.8205, 29.3748) (35.7242, 30.2784) (35.7242, 31.7435) (34.8205, 32.6469) knots 0 0 0 0 1 1 1 1
  line L1061 (34.8205, 29.3748) -> (35.7242, 30.2784) construction
  line L1062 (35.7242, 30.2784) -> (35.7242, 31.7435) construction
  line L1063 (35.7242, 31.7435) -> (34.8205, 32.6469) construction
  line L1064 (34.8205, 32.6469) -> (32.6391, 34.8284)
  spline S157 degree 3 poles (32.6391, 34.8284) (31.7354, 35.732) (30.2706, 35.732) (29.3669, 34.8284) knots 2 2 2 2 3 3 3 3
  line L1065 (32.6391, 34.8284) -> (31.7354, 35.732) construction
  line L1066 (31.7354, 35.732) -> (30.2706, 35.732) construction
  line L1067 (30.2706, 35.732) -> (29.3669, 34.8284) construction
  line L1068 (29.3669, 34.8284) -> (21.7319, 27.1933)
  spline S158 degree 3 poles (21.7319, 27.1933) (20.8283, 26.2899) (20.8283, 24.8248) (21.7319, 23.9212) knots 4 4 4 4 5 5 5 5
  line L1069 (21.7319, 27.1933) -> (20.8283, 26.2899) construction
  line L1070 (20.8283, 26.2899) -> (20.8283, 24.8248) construction
  line L1071 (20.8283, 24.8248) -> (21.7319, 23.9212) construction
  line L1072 (21.7319, 23.9212) -> (23.9134, 21.7398)
  spline S159 degree 3 poles (23.9134, 21.7398) (24.817, 20.8363) (26.2819, 20.8363) (27.1855, 21.7398) knots 6 6 6 6 7 7 7 7
  line L1073 (23.9134, 21.7398) -> (24.817, 20.8363) construction
  line L1074 (24.817, 20.8363) -> (26.2819, 20.8363) construction
  line L1075 (26.2819, 20.8363) -> (27.1855, 21.7398) construction
  line L1076 (27.1855, 21.7398) -> (34.8205, 29.3748)
  spline S160 degree 3 poles (48.9626, 43.5169) (49.8663, 44.4205) (49.8663, 45.8856) (48.9626, 46.789) knots 0 0 0 0 1 1 1 1
  line L1077 (48.9626, 43.5169) -> (49.8663, 44.4205) construction
  line L1078 (49.8663, 44.4205) -> (49.8663, 45.8856) construction
  line L1079 (49.8663, 45.8856) -> (48.9626, 46.789) construction
  line L1080 (48.9626, 46.789) -> (46.7812, 48.9705)
  spline S161 degree 3 poles (46.7812, 48.9705) (45.8776, 49.8741) (44.4127, 49.8741) (43.5091, 48.9705) knots 2 2 2 2 3 3 3 3
  line L1081 (46.7812, 48.9705) -> (45.8776, 49.8741) construction
  line L1082 (45.8776, 49.8741) -> (44.4127, 49.8741) construction
  line L1083 (44.4127, 49.8741) -> (43.5091, 48.9705) construction
  line L1084 (43.5091, 48.9705) -> (35.874, 41.3355)
  spline S162 degree 3 poles (35.874, 41.3355) (34.9704, 40.432) (34.9704, 38.967) (35.874, 38.0633) knots 4 4 4 4 5 5 5 5
  line L1085 (35.874, 41.3355) -> (34.9704, 40.432) construction
  line L1086 (34.9704, 40.432) -> (34.9704, 38.967) construction
  line L1087 (34.9704, 38.967) -> (35.874, 38.0633) construction
  line L1088 (35.874, 38.0633) -> (38.0555, 35.882)
  spline S163 degree 3 poles (38.0555, 35.882) (38.9591, 34.9784) (40.424, 34.9784) (41.3276, 35.882) knots 6 6 6 6 7 7 7 7
  line L1089 (38.0555, 35.882) -> (38.9591, 34.9784) construction
  line L1090 (38.9591, 34.9784) -> (40.424, 34.9784) construction
  line L1091 (40.424, 34.9784) -> (41.3276, 35.882) construction
  line L1092 (41.3276, 35.882) -> (48.9626, 43.5169)
  line L1093 (-63.1111, 61.0099) -> (-63.1003, 61.2245)
  line L1094 (-63.1003, 61.2245) -> (-63.0684, 61.4331)
  line L1095 (-63.0684, 61.4331) -> (-63.0167, 61.6343)
  line L1096 (-63.0167, 61.6343) -> (-62.9461, 61.8272)
  line L1097 (-62.9461, 61.8272) -> (-62.8577, 62.0109)
  line L1098 (-62.8577, 62.0109) -> (-62.7525, 62.184)
  line L1099 (-62.7525, 62.184) -> (-62.6316, 62.3455)
  line L1100 (-62.6316, 62.3455) -> (-62.496, 62.4947)
  line L1101 (-62.496, 62.4947) -> (-62.347, 62.6303)
  line L1102 (-62.347, 62.6303) -> (-62.1853, 62.7512)
  line L1103 (-62.1853, 62.7512) -> (-62.0121, 62.8565)
  line L1104 (-62.0121, 62.8565) -> (-61.8285, 62.9448)
  line L1105 (-61.8285, 62.9448) -> (-61.6356, 63.0154)
  line L1106 (-61.6356, 63.0154) -> (-61.4344, 63.0671)
  line L1107 (-61.4344, 63.0671) -> (-61.2258, 63.099)
  line L1108 (-61.2258, 63.099) -> (-61.0112, 63.1098)
  line L1109 (-61.0112, 63.1098) -> (-60.7964, 63.099)
  line L1110 (-60.7964, 63.099) -> (-60.5879, 63.0671)
  line L1111 (-60.5879, 63.0671) -> (-60.3866, 63.0154)
  line L1112 (-60.3866, 63.0154) -> (-60.1937, 62.9448)
  line L1113 (-60.1937, 62.9448) -> (-60.0102, 62.8565)
  line L1114 (-60.0102, 62.8565) -> (-59.8371, 62.7512)
  line L1115 (-59.8371, 62.7512) -> (-59.6753, 62.6303)
  line L1116 (-59.6753, 62.6303) -> (-59.5262, 62.4947)
  line L1117 (-59.5262, 62.4947) -> (-59.3906, 62.3455)
  line L1118 (-59.3906, 62.3455) -> (-59.2699, 62.184)
  line L1119 (-59.2699, 62.184) -> (-59.1646, 62.0109)
  line L1120 (-59.1646, 62.0109) -> (-59.0762, 61.8272)
  line L1121 (-59.0762, 61.8272) -> (-59.0056, 61.6343)
  line L1122 (-59.0056, 61.6343) -> (-58.9538, 61.4331)
  line L1123 (-58.9538, 61.4331) -> (-58.9219, 61.2245)
  line L1124 (-58.9219, 61.2245) -> (-58.9112, 61.0099)
  line L1125 (-58.9112, 61.0099) -> (-58.9219, 60.7951)
  line L1126 (-58.9219, 60.7951) -> (-58.9538, 60.5867)
  line L1127 (-58.9538, 60.5867) -> (-59.0056, 60.3853)
  line L1128 (-59.0056, 60.3853) -> (-59.0762, 60.1924)
  line L1129 (-59.0762, 60.1924) -> (-59.1646, 60.0087)
  line L1130 (-59.1646, 60.0087) -> (-59.2699, 59.8356)
  line L1131 (-59.2699, 59.8356) -> (-59.3906, 59.674)
  line L1132 (-59.3906, 59.674) -> (-59.5262, 59.5249)
  line L1133 (-59.5262, 59.5249) -> (-59.6753, 59.3893)
  line L1134 (-59.6753, 59.3893) -> (-59.8371, 59.2684)
  line L1135 (-59.8371, 59.2684) -> (-60.0102, 59.1633)
  line L1136 (-60.0102, 59.1633) -> (-60.1937, 59.0748)
  line L1137 (-60.1937, 59.0748) -> (-60.3866, 59.0042)
  line L1138 (-60.3866, 59.0042) -> (-60.5879, 58.9525)
  line L1139 (-60.5879, 58.9525) -> (-60.7964, 58.9206)
  line L1140 (-60.7964, 58.9206) -> (-61.0112, 58.9098)
  line L1141 (-61.0112, 58.9098) -> (-61.2258, 58.9206)
  line L1142 (-61.2258, 58.9206) -> (-61.4344, 58.9525)
  line L1143 (-61.4344, 58.9525) -> (-61.6356, 59.0042)
  line L1144 (-61.6356, 59.0042) -> (-61.8285, 59.0748)
  line L1145 (-61.8285, 59.0748) -> (-62.0121, 59.1633)
  line L1146 (-62.0121, 59.1633) -> (-62.1853, 59.2684)
  line L1147 (-62.1853, 59.2684) -> (-62.347, 59.3893)
  line L1148 (-62.347, 59.3893) -> (-62.496, 59.5249)
  line L1149 (-62.496, 59.5249) -> (-62.6316, 59.674)
  line L1150 (-62.6316, 59.674) -> (-62.7525, 59.8356)
  line L1151 (-62.7525, 59.8356) -> (-62.8577, 60.0087)
  line L1152 (-62.8577, 60.0087) -> (-62.9461, 60.1924)
  line L1153 (-62.9461, 60.1924) -> (-63.0167, 60.3853)
  line L1154 (-63.0167, 60.3853) -> (-63.0684, 60.5867)
  line L1155 (-63.0684, 60.5867) -> (-63.1003, 60.7951)
  line L1156 (-63.1003, 60.7951) -> (-63.1111, 61.0099)
  line L1157 (58.8973, 61.0099) -> (58.9079, 61.2245)
  line L1158 (58.9079, 61.2245) -> (58.94, 61.4331)
  line L1159 (58.94, 61.4331) -> (58.9917, 61.6343)
  line L1160 (58.9917, 61.6343) -> (59.0623, 61.8272)
  line L1161 (59.0623, 61.8272) -> (59.1505, 62.0109)
  line L1162 (59.1505, 62.0109) -> (59.2559, 62.184)
  line L1163 (59.2559, 62.184) -> (59.3768, 62.3455)
  line L1164 (59.3768, 62.3455) -> (59.5122, 62.4947)
  line L1165 (59.5122, 62.4947) -> (59.6614, 62.6303)
  line L1166 (59.6614, 62.6303) -> (59.823, 62.7512)
  line L1167 (59.823, 62.7512) -> (59.9963, 62.8565)
  line L1168 (59.9963, 62.8565) -> (60.1799, 62.9448)
  line L1169 (60.1799, 62.9448) -> (60.3728, 63.0154)
  line L1170 (60.3728, 63.0154) -> (60.574, 63.0671)
  line L1171 (60.574, 63.0671) -> (60.7824, 63.099)
  line L1172 (60.7824, 63.099) -> (60.9971, 63.1098)
  line L1173 (60.9971, 63.1098) -> (61.212, 63.099)
  line L1174 (61.212, 63.099) -> (61.4205, 63.0671)
  line L1175 (61.4205, 63.0671) -> (61.6216, 63.0154)
  line L1176 (61.6216, 63.0154) -> (61.8146, 62.9448)
  line L1177 (61.8146, 62.9448) -> (61.9982, 62.8565)
  line L1178 (61.9982, 62.8565) -> (62.1711, 62.7512)
  line L1179 (62.1711, 62.7512) -> (62.3331, 62.6303)
  line L1180 (62.3331, 62.6303) -> (62.4822, 62.4947)
  line L1181 (62.4822, 62.4947) -> (62.6176, 62.3455)
  line L1182 (62.6176, 62.3455) -> (62.7385, 62.184)
  line L1183 (62.7385, 62.184) -> (62.8436, 62.0109)
  line L1184 (62.8436, 62.0109) -> (62.9322, 61.8272)
  line L1185 (62.9322, 61.8272) -> (63.0028, 61.6343)
  line L1186 (63.0028, 61.6343) -> (63.0545, 61.4331)
  line L1187 (63.0545, 61.4331) -> (63.0862, 61.2245)
  line L1188 (63.0862, 61.2245) -> (63.0972, 61.0099)
  line L1189 (63.0972, 61.0099) -> (63.0862, 60.7951)
  line L1190 (63.0862, 60.7951) -> (63.0545, 60.5867)
  line L1191 (63.0545, 60.5867) -> (63.0028, 60.3853)
  line L1192 (63.0028, 60.3853) -> (62.9322, 60.1924)
  line L1193 (62.9322, 60.1924) -> (62.8436, 60.0087)
  line L1194 (62.8436, 60.0087) -> (62.7385, 59.8356)
  line L1195 (62.7385, 59.8356) -> (62.6176, 59.674)
  line L1196 (62.6176, 59.674) -> (62.4822, 59.5249)
  line L1197 (62.4822, 59.5249) -> (62.3331, 59.3893)
  line L1198 (62.3331, 59.3893) -> (62.1711, 59.2684)
  line L1199 (62.1711, 59.2684) -> (61.9982, 59.1633)
  line L1200 (61.9982, 59.1633) -> (61.8146, 59.0748)
  line L1201 (61.8146, 59.0748) -> (61.6216, 59.0042)
  line L1202 (61.6216, 59.0042) -> (61.4205, 58.9525)
  line L1203 (61.4205, 58.9525) -> (61.212, 58.9206)
  line L1204 (61.212, 58.9206) -> (60.9971, 58.9098)
  line L1205 (60.9971, 58.9098) -> (60.7824, 58.9206)
  line L1206 (60.7824, 58.9206) -> (60.574, 58.9525)
  line L1207 (60.574, 58.9525) -> (60.3728, 59.0042)
  line L1208 (60.3728, 59.0042) -> (60.1799, 59.0748)
  line L1209 (60.1799, 59.0748) -> (59.9963, 59.1633)
  line L1210 (59.9963, 59.1633) -> (59.823, 59.2684)
  line L1211 (59.823, 59.2684) -> (59.6614, 59.3893)
  line L1212 (59.6614, 59.3893) -> (59.5122, 59.5249)
  line L1213 (59.5122, 59.5249) -> (59.3768, 59.674)
  line L1214 (59.3768, 59.674) -> (59.2559, 59.8356)
  line L1215 (59.2559, 59.8356) -> (59.1505, 60.0087)
  line L1216 (59.1505, 60.0087) -> (59.0623, 60.1924)
  line L1217 (59.0623, 60.1924) -> (58.9917, 60.3853)
  line L1218 (58.9917, 60.3853) -> (58.94, 60.5867)
  line L1219 (58.94, 60.5867) -> (58.9079, 60.7951)
  line L1220 (58.9079, 60.7951) -> (58.8973, 61.0099)
  line L1221 (58.8973, -60.9985) -> (58.9079, -60.7839)
  line L1222 (58.9079, -60.7839) -> (58.94, -60.5751)
  line L1223 (58.94, -60.5751) -> (58.9917, -60.3739)
  line L1224 (58.9917, -60.3739) -> (59.0623, -60.181)
  line L1225 (59.0623, -60.181) -> (59.1505, -59.9974)
  line L1226 (59.1505, -59.9974) -> (59.2559, -59.8244)
  line L1227 (59.2559, -59.8244) -> (59.3768, -59.6629)
  line L1228 (59.3768, -59.6629) -> (59.5122, -59.5137)
  line L1229 (59.5122, -59.5137) -> (59.6614, -59.3779)
  line L1230 (59.6614, -59.3779) -> (59.823, -59.257)
  line L1231 (59.823, -59.257) -> (59.9963, -59.1519)
  line L1232 (59.9963, -59.1519) -> (60.1799, -59.0634)
  line L1233 (60.1799, -59.0634) -> (60.3728, -58.9928)
  line L1234 (60.3728, -58.9928) -> (60.574, -58.9411)
  line L1235 (60.574, -58.9411) -> (60.7824, -58.9094)
  line L1236 (60.7824, -58.9094) -> (60.9971, -58.8984)
  line L1237 (60.9971, -58.8984) -> (61.212, -58.9094)
  line L1238 (61.212, -58.9094) -> (61.4205, -58.9411)
  line L1239 (61.4205, -58.9411) -> (61.6216, -58.9928)
  line L1240 (61.6216, -58.9928) -> (61.8146, -59.0634)
  line L1241 (61.8146, -59.0634) -> (61.9982, -59.1519)
  line L1242 (61.9982, -59.1519) -> (62.1711, -59.257)
  line L1243 (62.1711, -59.257) -> (62.3331, -59.3779)
  line L1244 (62.3331, -59.3779) -> (62.4822, -59.5137)
  line L1245 (62.4822, -59.5137) -> (62.6176, -59.6629)
  line L1246 (62.6176, -59.6629) -> (62.7385, -59.8244)
  line L1247 (62.7385, -59.8244) -> (62.8436, -59.9974)
  line L1248 (62.8436, -59.9974) -> (62.9322, -60.181)
  line L1249 (62.9322, -60.181) -> (63.0028, -60.3739)
  line L1250 (63.0028, -60.3739) -> (63.0545, -60.5751)
  line L1251 (63.0545, -60.5751) -> (63.0862, -60.7839)
  line L1252 (63.0862, -60.7839) -> (63.0972, -60.9985)
  line L1253 (63.0972, -60.9985) -> (63.0862, -61.2131)
  line L1254 (63.0862, -61.2131) -> (63.0545, -61.4216)
  line L1255 (63.0545, -61.4216) -> (63.0028, -61.6231)
  line L1256 (63.0028, -61.6231) -> (62.9322, -61.816)
  line L1257 (62.9322, -61.816) -> (62.8436, -61.9993)
  line L1258 (62.8436, -61.9993) -> (62.7385, -62.1726)
  line L1259 (62.7385, -62.1726) -> (62.6176, -62.3342)
  line L1260 (62.6176, -62.3342) -> (62.4822, -62.4834)
  line L1261 (62.4822, -62.4834) -> (62.3331, -62.6191)
  line L1262 (62.3331, -62.6191) -> (62.1711, -62.74)
  line L1263 (62.1711, -62.74) -> (61.9982, -62.8451)
  line L1264 (61.9982, -62.8451) -> (61.8146, -62.9336)
  line L1265 (61.8146, -62.9336) -> (61.6216, -63.0039)
  line L1266 (61.6216, -63.0039) -> (61.4205, -63.0559)
  line L1267 (61.4205, -63.0559) -> (61.212, -63.0876)
  line L1268 (61.212, -63.0876) -> (60.9971, -63.0986)
  line L1269 (60.9971, -63.0986) -> (60.7824, -63.0876)
  line L1270 (60.7824, -63.0876) -> (60.574, -63.0559)
  line L1271 (60.574, -63.0559) -> (60.3728, -63.0039)
  line L1272 (60.3728, -63.0039) -> (60.1799, -62.9336)
  line L1273 (60.1799, -62.9336) -> (59.9963, -62.8451)
  line L1274 (59.9963, -62.8451) -> (59.823, -62.74)
  line L1275 (59.823, -62.74) -> (59.6614, -62.6191)
  line L1276 (59.6614, -62.6191) -> (59.5122, -62.4834)
  line L1277 (59.5122, -62.4834) -> (59.3768, -62.3342)
  line L1278 (59.3768, -62.3342) -> (59.2559, -62.1726)
  line L1279 (59.2559, -62.1726) -> (59.1505, -61.9993)
  line L1280 (59.1505, -61.9993) -> (59.0623, -61.816)
  line L1281 (59.0623, -61.816) -> (58.9917, -61.6231)
  line L1282 (58.9917, -61.6231) -> (58.94, -61.4216)
  line L1283 (58.94, -61.4216) -> (58.9079, -61.2131)
  line L1284 (58.9079, -61.2131) -> (58.8973, -60.9985)
  line L1285 (-63.1017, -60.9985) -> (-63.0908, -60.7839)
  line L1286 (-63.0908, -60.7839) -> (-63.0589, -60.5751)
  line L1287 (-63.0589, -60.5751) -> (-63.0073, -60.3739)
  line L1288 (-63.0073, -60.3739) -> (-62.9366, -60.181)
  line L1289 (-62.9366, -60.181) -> (-62.8483, -59.9974)
  line L1290 (-62.8483, -59.9974) -> (-62.743, -59.8244)
  line L1291 (-62.743, -59.8244) -> (-62.6221, -59.6629)
  line L1292 (-62.6221, -59.6629) -> (-62.4865, -59.5137)
  line L1293 (-62.4865, -59.5137) -> (-62.3375, -59.3779)
  line L1294 (-62.3375, -59.3779) -> (-62.1758, -59.257)
  line L1295 (-62.1758, -59.257) -> (-62.0027, -59.1519)
  line L1296 (-62.0027, -59.1519) -> (-61.8191, -59.0634)
  line L1297 (-61.8191, -59.0634) -> (-61.6261, -58.9928)
  line L1298 (-61.6261, -58.9928) -> (-61.4249, -58.9411)
  line L1299 (-61.4249, -58.9411) -> (-61.2163, -58.9094)
  line L1300 (-61.2163, -58.9094) -> (-61.0017, -58.8984)
  line L1301 (-61.0017, -58.8984) -> (-60.7869, -58.9094)
  line L1302 (-60.7869, -58.9094) -> (-60.5785, -58.9411)
  line L1303 (-60.5785, -58.9411) -> (-60.3773, -58.9928)
  line L1304 (-60.3773, -58.9928) -> (-60.1844, -59.0634)
  line L1305 (-60.1844, -59.0634) -> (-60.0007, -59.1519)
  line L1306 (-60.0007, -59.1519) -> (-59.8276, -59.257)
  line L1307 (-59.8276, -59.257) -> (-59.6659, -59.3779)
  line L1308 (-59.6659, -59.3779) -> (-59.5167, -59.5137)
  line L1309 (-59.5167, -59.5137) -> (-59.3813, -59.6629)
  line L1310 (-59.3813, -59.6629) -> (-59.2604, -59.8244)
  line L1311 (-59.2604, -59.8244) -> (-59.1551, -59.9974)
  line L1312 (-59.1551, -59.9974) -> (-59.0668, -60.181)
  line L1313 (-59.0668, -60.181) -> (-58.9961, -60.3739)
  line L1314 (-58.9961, -60.3739) -> (-58.9443, -60.5751)
  line L1315 (-58.9443, -60.5751) -> (-58.9126, -60.7839)
  line L1316 (-58.9126, -60.7839) -> (-58.9017, -60.9985)
  line L1317 (-58.9017, -60.9985) -> (-58.9126, -61.2131)
  line L1318 (-58.9126, -61.2131) -> (-58.9443, -61.4216)
  line L1319 (-58.9443, -61.4216) -> (-58.9961, -61.6231)
  line L1320 (-58.9961, -61.6231) -> (-59.0668, -61.816)
  line L1321 (-59.0668, -61.816) -> (-59.1551, -61.9993)
  line L1322 (-59.1551, -61.9993) -> (-59.2604, -62.1726)
  line L1323 (-59.2604, -62.1726) -> (-59.3813, -62.3342)
  line L1324 (-59.3813, -62.3342) -> (-59.5167, -62.4834)